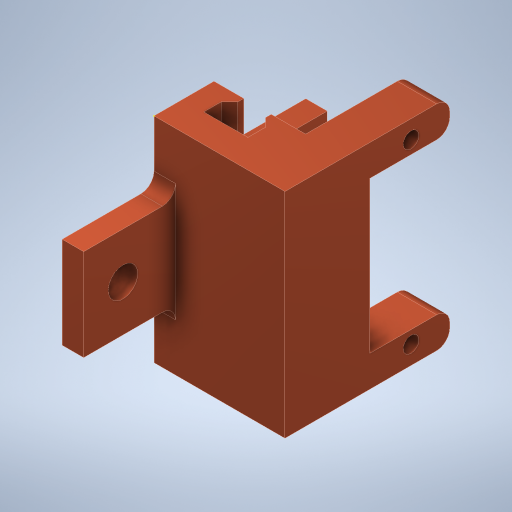
# Autodesk Inventor part: Motor_holder_double
Saved by Autodesk Inventor 2024.2 (Build 282272000, 272)
## iProperties
Created: 2025-06-02
Part Number: Motor_holder_double
Material: Měď
Document SubType Name: Modeling
Designer: Elite
Density: 8.94 g/cm^3
Appearance: Měď – satén
Mass: 95.1556 g
Surface Area: 50.1955 cm^2
Volume: 10.6438 cm^3
Author: Elite
Autodesk Inventor part; units mm, degrees
ref_plane "YZ Plane" through (0, 0, 0) normal (1, 0, 0) x (0, 1, 0)
ref_plane "XZ Plane" through (0, 0, 0) normal (0, 1, 0) x (-1, 0, 0)
ref_plane "XY Plane" through (0, 0, 0) normal (0, 0, 1) x (1, 0, 0)
sketch "Náčrt1" plane through (0, 0, 0) normal (0, 0, 1) x (1, 0, 0)
  line L0 (13.97, 23.865) -> (13.97, 9.144)
  line L1 (0, 9.144) -> (0, 0)
  line L2 (4.5409, 9.144) -> (0, 9.144)
  line L3 (4.5409, 8.255) -> (4.5409, 9.144)
  line L4 (3.2709, 6.985) -> (4.5409, 8.255)
  line L5 (3.2709, 4.318) -> (3.2709, 6.985)
  line L6 (8.7319, 9.144) -> (8.7319, 8.255)
  line L7 (13.97, 9.144) -> (8.7319, 9.144)
  line L8 (8.7319, 8.255) -> (10.0019, 6.985)
  line L9 (10.0019, 6.985) -> (10.0019, 4.318)
  line L10 (10.0019, 4.318) -> (3.2709, 4.318)
  line L11 (0, 0) -> (19.97, 0)
  line L12 (13.97, 22.5956) -> (13.97, 25.1349)
  line L13 (13.97, 20.4353) -> (13.97, 18.035)
  line L14 (13.97, 25.1349) -> (19.97, 25.1349)
  line L15 (19.97, 25.1349) -> (19.97, 0)
  constraints: 32 end point, 1 horizontal, 1 vertical
extrude "Vysunutí1" add sketch "Náčrt1" against normal blind 32.6
sketch "Náčrt2" plane through (19.97, 0, 0) normal (1, 0, 0) x (0, 0, -1)
  line L0 (0, 25.1349) -> (32.6, 25.1349) projected
  line L1 (16.3, 25.1349) -> (4.746, 25.1349)
  line L2 (4.746, 25.1349) -> (4.746, 12.9539)
  line L3 (16.3, 25.1349) -> (27.854, 25.1349)
  line L4 (27.854, 25.1349) -> (27.854, 12.9539)
  line L5 (27.854, 12.9539) -> (4.746, 12.9539)
  circle A0 centre (2.8, 19.2349) radius 1.2
  line L6 (16.3, 25.1349) -> (16.3, 15.9225)
  circle A1 centre (29.8, 19.2349) radius 1.2
  point P0 (0, 0)
  point P1 (4.746, 19.0444)
  dimension "d2" = 11.554
  dimension "d3" = 12.181
  dimension "d4" = 11.554
  dimension "d7" = 2.4
  dimension "d8" = 5.9
  dimension "d9" = 1.946
  constraints: 12 end point, 3 perpendicular, 2 centre point, 2 midpoint, 2 point on line, 1 symmetric about line, 1 vertical, 1 other
  measures "d2" distance of L1.start L1.end
  measures "d3" distance of L1.end L2.end
  measures "d4" distance of L1.start L3.end
  measures "d7" diameter of A0
  measures "d8" distance from line of L0 A0.centre
  measures "d9" horizontal distance of point (4.746, 19.044) A0.centre
extrude "Vysunutí2" cut sketch "Náčrt2" against normal blind 32.6 contours L0 L4 L5 L2
extrude "Vysunutí3" cut sketch "Náčrt2" against normal blind 32.6 contours A0 | A1
fillet "Zaoblení1" radius 2 4 edges at (16.97, 25.1349, 0) (16.97, 25.1349, -4.746) (16.97, 25.1349, -27.854) (16.97, 25.1349, -32.6)
sketch "Náčrt3" plane through (0, 0, 0) normal (0, -1, 0) x (1, 0, 0)
  point P0 (0, 0)
sketch "Náčrt8" plane through (0, 0, 0) normal (-1, 0, 0) x (0, 0, 1)
  line L0 (0, 9.144) -> (-32.6, 9.144) projected
  line L1 (0, 0) -> (-32.6, 0) projected
  circle A0 centre (-16.3, 17.144) radius 2.25
  line L2 (-23.3, 9.144) -> (-9.3, 9.144)
  line L3 (-9.3, 9.144) -> (-9.3, 23.144)
  line L4 (-9.3, 23.144) -> (-23.3, 23.144)
  line L5 (-23.3, 23.144) -> (-23.3, 9.144)
  line L6 (0, 9.144) -> (0, 0) projected
  line L7 (0, 9.144) -> (0, 0)
  line L8 (0, 4.572) -> (9.3918, 4.572)
  circle A1 centre (-16.3, -8) radius 2.25
  line L9 (-23.3, 0) -> (-9.3, 0)
  line L10 (-9.3, 0) -> (-9.3, -14)
  line L11 (-9.3, -14) -> (-23.3, -14)
  line L12 (-23.3, -14) -> (-23.3, 0)
  point P0 (-16.3, 9.144)
  point P1 (-16.3, 9.144)
  point P2 (-16.3, 0)
  point P3 (-16.3, 0)
  dimension "d35" = 4.5
  dimension "d36" = 8
  dimension "k" = 14
  dimension "d42" = 14
  dimension "d43" = 7
  dimension "d44" = 7
  constraints: 20 end point, 7 symmetric about line, 3 equal length, 3 midpoint, 2 centre point, 2 horizontal, 1 perpendicular, 1 point on line, 1 other
  measures "d35" diameter of A0
  measures "d36" distance of point (-16.3, 9.144) A0.centre
  measures "k" distance of L4.end L3.end
  measures "d42" distance of L4.end L2.start
  measures "d43" distance from line of L5 A0.centre
  measures "d44" distance of L2.end point (-16.3, 9.144)
extrude "Vysunutí7" add sketch "Náčrt8" against normal up to surface (3.2709 mm away)
fillet "Zaoblení2" radius 2 4 edges at (1.6355, 9.144, -9.3) (1.6355, 0, -9.3) (1.6355, 9.144, -23.3) (1.6355, 0, -23.3)
equation "\"d43\" = 0.5 * k"
equation "\"d44\" = 0.5 * k"
